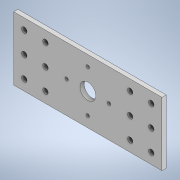
# Autodesk Inventor part: Motor Mount Long
Saved by Autodesk Inventor 2020 (Build 240168000, 168)
## iProperties
Created: 2020-02-11
Part Number: Motor Mount Long
Material: Generic
Document SubType Name: Modeling
Designer: 339294
Density: 1 g/cm^3
Appearance: Default
Author: 339294
Autodesk Inventor part; units mm, degrees
ref_plane "YZ Plane" through (0, 0, 0) normal (1, 0, 0) x (0, 1, 0)
ref_plane "XZ Plane" through (0, 0, 0) normal (0, 1, 0) x (-1, 0, 0)
ref_plane "XY Plane" through (0, 0, 0) normal (0, 0, 1) x (1, 0, 0)
sketch "Sketch1" plane through (0, 0, 0) normal (0, 0, 1) x (1, 0, 0)
  line L0 (0, 0) -> (177.8, 0)
  line L1 (177.8, 0) -> (177.8, 76.2)
  line L2 (177.8, 76.2) -> (0, 76.2)
  line L3 (0, 76.2) -> (0, 0)
  circle A0 centre (88.9, 38.1) radius 9.525
  circle A1 centre (88.9, 63.5) radius 2.0193
  circle A2 centre (63.5, 38.1) radius 2.0193
  circle A3 centre (88.9, 12.7) radius 2.0193
  circle A4 centre (114.3, 38.1) radius 2.0193
  circle A5 centre (12.7, 63.5) radius 3.2512
  circle A6 centre (12.7, 38.1) radius 3.2512
  circle A7 centre (12.7, 12.7) radius 3.2512
  circle A8 centre (38.1, 63.5) radius 3.2512
  circle A9 centre (38.1, 38.1) radius 3.2512
  circle A10 centre (38.1, 12.7) radius 3.2512
  circle A11 centre (165.1, 63.5) radius 3.2512
  circle A12 centre (165.1, 38.1) radius 3.2512
  circle A13 centre (165.1, 12.7) radius 3.2512
  circle A14 centre (139.7, 63.5) radius 3.2512
  circle A15 centre (139.7, 38.1) radius 3.2512
  circle A16 centre (139.7, 12.7) radius 3.2512
  dimension "d0" = 177.8
  dimension "d1" = 76.2
  dimension "d2" = 19.05
  dimension "d3" = 38.1
  dimension "d4" = 88.9
  dimension "d5" = 4.0386
  dimension "d6" = 25.4
  dimension "d7" = 88.9
  dimension "d8" = 4.0386
  dimension "d9" = 25.4
  dimension "d10" = 38.1
  dimension "d13" = 50.8
  dimension "d20" = 50.8
  dimension "d25" = 6.5024
  dimension "d26" = 12.7
  dimension "d27" = 12.7
  dimension "d30" = 25.4
  dimension "d39" = 25.4
  dimension "d48" = 127
  dimension "d55" = 25.4
  constraints: 17 centre point, 8 end point, 5 horizontal, 2 parallel, 2 vertical, 1 perpendicular, 26 other
  measures "d0" distance of L2.end L1.end
  measures "d1" distance of L1.end L0.end
  measures "d2" diameter of A0
  measures "d3" distance from line of L2 A0.centre
  measures "d4" distance from line of L1 A0.centre
  measures "d5" diameter of A1
  measures "d6" distance of A0.centre A1.centre
  measures "d7" distance from line of L1 A1.centre
  measures "d8" diameter of A2
  measures "d9" distance of A0.centre A2.centre
  measures "d10" distance from line of L2 A2.centre
  measures "d13" distance of A1.centre A3.centre
  measures "d20" distance of A2.centre A4.centre
  measures "d25" diameter of A5
  measures "d26" distance from line of L2 A5.centre
  measures "d27" distance from line of L3 A5.centre
  measures "d30" distance of A5.centre A6.centre
  measures "d39" distance of A5.centre A8.centre
  measures "d48" distance of A8.centre A11.centre
  measures "d55" distance of A11.centre A14.centre
extrude "Extrusion3" add sketch "Sketch1" along normal blind 5.08
equation "\"d7\" = d4"
equation "\"d8\" = d5"
equation "\"d9\" = d6"
equation "\"d10\" = d3"
body "Solid3"
